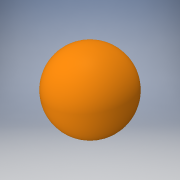
# Autodesk Inventor part: Sphere
Saved by Autodesk Inventor 2016 (Build 200138000, 138)
## iProperties
Created: 2017-02-09
Part Number: Sphere
Material: Generic
Document SubType Name: Modeling
Designer: Evan Phil George
Density: 1 g/cm^3
Appearance: Default
Author: Evan Phil George
Autodesk Inventor part; units mm, degrees
ref_plane "YZ Plane" through (0, 0, 0) normal (1, 0, 0) x (0, 1, 0)
ref_plane "XZ Plane" through (0, 0, 0) normal (0, 1, 0) x (-1, 0, 0)
ref_plane "XY Plane" through (0, 0, 0) normal (0, 0, 1) x (1, 0, 0)
sketch "Sketch1" plane through (0, 0, 0) normal (1, 0, 0) x (0, 1, 0)
  arc A0 (119.3, 0) -> (-119.3, 0) centre (0, 0) ccw
  arc A1 (117.3, 0) -> (-117.3, 0) centre (0, 0) ccw
  line L0 (0, 0) -> (117.3, 0)
  line L1 (0, 0) -> (-117.3, 0)
  line L2 (117.3, 0) -> (119.3, 0)
  line L3 (-117.3, 0) -> (-119.3, 0)
  dimension "d0" = 238.6
  dimension "d1" = 234.6
  constraints: 8 end point, 4 horizontal, 4 point on circle, 2 centre point, 2 coincident
  measures "d0" diameter of A0
  measures "d1" diameter of A1
revolve "Revolution1" add sketch "Sketch1" angle 360 about axis through (0, 0, 0) along (0, 1, 0) contours L2 A1 L3 A0
body "Solid1"
